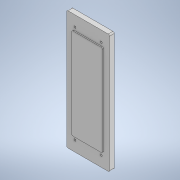
# Autodesk Inventor part: PanelJig
Saved by Autodesk Inventor 2021 (Build 250183000, 183)
## iProperties
Created: 2020-07-25
Part Number: PanelJig
Material: Generic
Document SubType Name: Modeling
Designer: CASE-SMALL2
Density: 1 g/cm^3
Appearance: Default
Author: CASE-SMALL2
Autodesk Inventor part; units mm, degrees
ref_plane "YZ Plane" through (0, 0, 0) normal (1, 0, 0) x (0, 1, 0)
ref_plane "XZ Plane" through (0, 0, 0) normal (0, 1, 0) x (-1, 0, 0)
ref_plane "XY Plane" through (0, 0, 0) normal (0, 0, 1) x (1, 0, 0)
sketch "Sketch1" plane through (0, 0, 0) normal (0, 0, 1) x (1, 0, 0)
  line L0 (-33.5, -93) -> (33.5, -93)
  line L1 (33.5, -93) -> (33.5, 93)
  line L2 (33.5, 93) -> (-33.5, 93)
  line L3 (-33.5, 93) -> (-33.5, -93)
  line L4 (-33.5, -93) -> (33.5, 93) construction
  line L5 (33.5, -93) -> (-33.5, 93) construction
  point P0 (0, 0)
  dimension "d0" = 67
  dimension "d1" = 186
  constraints: 12 end point, 2 midpoint, 2 parallel, 1 horizontal, 1 perpendicular
  measures "d0" distance between parallel lines of L3 L1
  measures "d1" distance between parallel lines of L0 L2
extrude "Extrusion1" add sketch "Sketch1" along normal blind 7.4
sketch "Sketch2" plane through (0, 0, 7.4) normal (0, 0, 1) x (1, 0, 0)
  line L0 (24, 71.3) -> (-24, 71.3)
  line L1 (-24, 71.3) -> (-24, -71.3)
  line L2 (-24, -71.3) -> (24, -71.3)
  line L3 (24, -71.3) -> (24, 71.3)
  line L4 (24, 71.3) -> (-24, -71.3) construction
  line L5 (-24, 71.3) -> (24, -71.3) construction
  point P0 (0, 0)
  dimension "d4" = 48
  dimension "d5" = 142.6
  constraints: 12 end point, 2 midpoint, 2 parallel, 1 horizontal, 1 perpendicular
  measures "d4" distance between parallel lines of L1 L3
  measures "d5" distance between parallel lines of L0 L2
extrude "Extrusion2" add sketch "Sketch2" along normal blind 1.6
fillet "Fillet1" radius 2 8 edges at (24, 71.3, 8.2) (-24, 71.3, 8.2) (-24, -71.3, 8.2) (24, -71.3, 8.2) (-33.5, 93, 3.7) (33.5, 93, 3.7) (-33.5, -93, 3.7) (33.5, -93, 3.7)
sketch "Sketch3" plane through (0, 0, 9) normal (0, 0, 1) x (1, 0, 0)
  circle A0 centre (-20.5, -76.5) radius 1.5
  line L0 (-46.9, 0) -> (46.9, 0) construction
  line L1 (0, -130.2) -> (0, 130.2) construction
  circle A1 centre (-20.5, 76.5) radius 1.5
  circle A2 centre (20.5, -76.5) radius 1.5
  circle A3 centre (20.5, 76.5) radius 1.5
  point P0 (0, 0)
  dimension "d9" = 3
  dimension "d10" = 41
  dimension "d11" = 153
  constraints: 4 centre point, 3 symmetric about line, 3 other
  measures "d9" diameter of A0
  measures "d10" distance of A2.centre A0.centre
  measures "d11" distance of A1.centre A0.centre
extrude "Extrusion3" cut sketch "Sketch3" against normal through all
body "Solid1"
